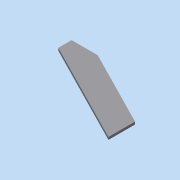
# Autodesk Inventor part: Angled foot
Saved by Autodesk Inventor 2016 (Build 200138000, 138)
## iProperties
Created: 2017-03-05
Part Number: Angled foot
Material: Generic
Document SubType Name: Modeling
Designer: Errrm
Density: 1 g/cm^3
Appearance: Default
Author: Errrm
Autodesk Inventor part; units mm, degrees
ref_plane "YZ Plane" through (0, 0, 0) normal (1, 0, 0) x (0, 1, 0)
ref_plane "XZ Plane" through (0, 0, 0) normal (0, 1, 0) x (-1, 0, 0)
ref_plane "XY Plane" through (0, 0, 0) normal (0, 0, 1) x (1, 0, 0)
sketch "Sketch1" plane through (0, 0, 0) normal (0, 0, 1) x (1, 0, 0)
  line L0 (25, -133.1907) -> (25, -79.0256)
  line L1 (25, -79.0256) -> (-129.9807, 0)
  line L2 (-183.0936, 0) -> (-183.0936, -27.0826)
  line L3 (-183.0936, -27.0826) -> (25, -133.1907)
  line L4 (-183.0936, 110) -> (-183.0936, -110) construction
  line L5 (25, 151) -> (-25, 151) construction
  line L6 (-25, 151) -> (-25, -151) construction
  line L7 (-25, -151) -> (25, -151) construction
  line L8 (25, -151) -> (25, 151) construction
  line L9 (-183.0936, 0) -> (-129.9807, 0)
  point P0 (0, 0)
  point P1 (25, -106.1081)
  constraints: 10 end point, 2 midpoint, 2 parallel, 1 horizontal, 1 point on line, 1 vertical
extrude "Extrusion1" add sketch "Sketch1" along normal blind 5
body "Solid1"
